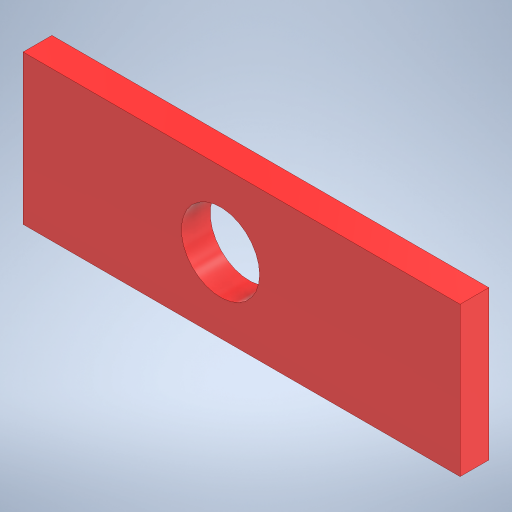
# Autodesk Inventor part: Grundplatte
Saved by Autodesk Inventor 2023 (Build 270158000, 158)
## iProperties
Created: 2023-01-17
Part Number: Grundplatte
Material: PBT-Kunststoff
Document SubType Name: Modeling
Designer: remoh
Density: 1.31 g/cm^3
Appearance: Hellrot
Author: remoh
Autodesk Inventor part; units mm, degrees
ref_plane "YZ Plane" through (0, 0, 0) normal (1, 0, 0) x (0, 1, 0)
ref_plane "XZ Plane" through (0, 0, 0) normal (0, 1, 0) x (-1, 0, 0)
ref_plane "XY Plane" through (0, 0, 0) normal (0, 0, 1) x (1, 0, 0)
sketch "Skizze1" plane through (0, 0, 0) normal (0, 0, 1) x (1, 0, 0)
  line L0 (0, 0) -> (24.3, 0)
  line L1 (24.3, 0) -> (24.3, -8.3)
  line L2 (24.3, -8.3) -> (0, -8.3)
  line L3 (0, -8.3) -> (0, 0)
  circle A0 centre (10.975, -4.15) radius 2.175
  dimension "d0" = 8.3
  dimension "d1" = 24.3
  dimension "d2" = 4.15
  dimension "d3" = 4.15
  dimension "d4" = 4.35
  dimension "d5" = 13.325
  constraints: 8 end point, 2 parallel, 1 centre point, 1 horizontal, 1 perpendicular
  measures "d0" distance of L2.end L0.start
  measures "d1" distance of L0.start L0.end
  measures "d2" distance from line of A0.centre L0
  measures "d3" distance from line of L2 A0.centre
  measures "d4" diameter of A0
  measures "d5" distance from line of A0.centre L1
extrude "Extrusion1" add sketch "Skizze1" along normal blind 1.6
equation "\"d2\" = d3"
